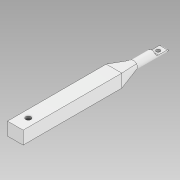
# Autodesk Inventor part: 3103_Bulb Arm_V2_Shortened
Saved by Autodesk Inventor 2020 (Build 240168000, 168)
## iProperties
Created: 2019-10-22
Part Number: 3103_Bulb Arm_V2_Shortened
Material: ABS Plastic
Document SubType Name: Modeling
Designer: RFLab
Density: 1.06 g/cm^3
Appearance: Smooth - White
Author: RFLab
Autodesk Inventor part; units mm, degrees
ref_plane "YZ Plane" through (0, 0, 0) normal (1, 0, 0) x (0, 1, 0)
ref_plane "XZ Plane" through (0, 0, 0) normal (0, 1, 0) x (-1, 0, 0)
ref_plane "XY Plane" through (0, 0, 0) normal (0, 0, 1) x (1, 0, 0)
sketch "Sketch8" plane through (0, 0, 0) normal (0, 0, 1) x (1, 0, 0)
  line L0 (-6, -5) -> (6, -5)
  line L1 (6, -5) -> (6, 5)
  line L2 (6, 5) -> (-6, 5)
  line L3 (-6, 5) -> (-6, -5)
  line L4 (-6, -5) -> (6, 5) construction
  line L5 (6, -5) -> (-6, 5) construction
  point P0 (0, 0)
  dimension "d41" = 12
  dimension "d42" = 10
  constraints: 12 end point, 2 midpoint, 2 parallel, 1 horizontal, 1 perpendicular
  measures "d41" distance of L2.end L1.end
  measures "d42" distance of L1.end L0.end
extrude "Extrusion8" add sketch "Sketch8" along normal blind 96
sketch "Sketch9" plane through (0, 0, 0) normal (0, 0, -1) x (-1, 0, 0)
  line L0 (6, 5) -> (6, -5) projected
  circle A0 centre (0, 0) radius 3
  point P0 (0, 0)
  point P1 (6, 0)
  dimension "d45" = 6
  constraints: 1 centre point, 1 horizontal alignment, 1 midpoint
  measures "d45" diameter of A0
extrude "Extrusion9" add sketch "Sketch9" along normal blind 59
sketch "Sketch10" plane through (0, 0, 0) normal (0, 0, -1) x (-1, 0, 0)
  line L0 (6, -5) -> (-6, -5) projected
  line L1 (6, 5) -> (6, -5) projected
  line L2 (-6, 5) -> (6, 5) projected
  line L3 (-6, -5) -> (-6, 5) projected
ref_plane "Work Plane2" through (0, 0, -15) normal (0, 0, -1) x (-1, 0, 0)
sketch "Sketch11" plane through (0, 0, -15) normal (0, 0, -1) x (-1, 0, 0)
  circle A0 centre (0, 0) radius 3 projected
  point P0 (0, 0)
loft "Loft3" add profiles "Sketch10", "Sketch11"
sketch "Sketch12" plane through (6, -5, 96) normal (1, 0, 0) x (0, 0, -1)
  line L0 (111, 8) -> (155, 8) projected
  line L1 (111, 2) -> (155, 2) projected
  line L2 (155, 2) -> (155, 8) projected
  line L3 (96, 10) -> (111, 6.9206) projected
  line L4 (111, 6.9206) -> (111, 6.9206) projected
  line L5 (96, 10) -> (111, 6.9206) projected
  line L6 (96, 0) -> (111, 3.0794) projected
  line L7 (111, 3.0794) -> (111, 3.0794) projected
  line L8 (96, 0) -> (111, 3.0794) projected
  line L9 (155, 8) -> (125, 8)
  line L10 (125, 8) -> (125, 5)
  line L11 (125, 5) -> (155, 5)
  line L12 (155, 5) -> (155, 8)
  line L13 (155, 5) -> (135, 5)
  line L14 (135, 5) -> (135, 2)
  line L15 (135, 2) -> (155, 2)
  line L16 (155, 2) -> (155, 5)
  point P0 (96, 5)
  dimension "d54" = 30
  dimension "d55" = 3
  dimension "d56" = 20
  constraints: 16 end point, 4 parallel, 2 horizontal, 2 perpendicular, 1 point on line
  measures "d54" distance of L11.end L10.end
  measures "d55" distance of L10.end L9.end
  measures "d56" distance of L15.end L14.end
extrude "Extrusion10" cut sketch "Sketch12" against normal blind 59
sketch "Sketch13" plane through (-3, 0, -39) normal (0, 1, 0) x (1, 0, 0)
  line L0 (6, 0) -> (0, 0) projected
  line L1 (0, -10) -> (6, -10) projected
  line L2 (3, -10) -> (3, 0)
  circle A0 centre (3, -5) radius 1.5
  point P0 (3, -39)
  dimension "d59" = 3
  constraints: 3 midpoint, 2 end point, 1 centre point
  measures "d59" diameter of A0
extrude "Extrusion11" cut sketch "Sketch13" against normal blind 59
fillet "Fillet2" radius 2 1 edges at (0, 0, -29)
fillet "Fillet3" radius 1 1 edges at (0, 0, -39)
sketch "Sketch14" plane through (-6, 5, 96) normal (0, 1, 0) x (1, 0, 0)
  line L0 (12, 0) -> (0, 0) projected
  line L1 (0, 0) -> (12, 0) projected
  line L2 (6, 0) -> (6, 96)
  point P0 (6, 10)
  point P1 (6, 30)
  dimension "d64" = 10
  dimension "d65" = 30
  constraints: 2 end point, 2 point on line, 1 midpoint, 1 perpendicular
  measures "d64" distance from line of L0 point (6, 10)
  measures "d65" distance from line of L0 point (6, 30)
hole "Hole1" at (0, 5, 86) at (0, 5, 66) direction (0, -1, 0) diameter 4 end through all
sketch "Sketch16" plane through (0, 0, 96) normal (0, 0, 1) x (1, 0, 0)
  line L0 (-6, -5) -> (6, -5) projected
  line L1 (6, -5) -> (6, 5) projected
  line L2 (6, 5) -> (-6, 5) projected
  line L3 (-6, 5) -> (-6, -5) projected
  point P0 (0, 0)
extrude "Extrusion12" cut sketch "Sketch16" against normal blind 20
body "Solid2"
